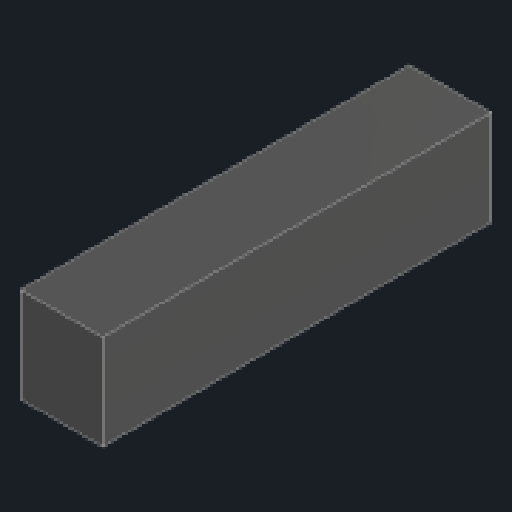
# Autodesk Inventor part: lipo2s450mah
Saved by Autodesk Inventor 2023 (Build 270158000, 158)
## iProperties
Created: 2024-05-25
Part Number: lipo2s450mah
Material: Generic
Document SubType Name: Modeling
Designer: szymo
Density: 2.33479 g/cm^3
Appearance: Dark Gray
Mass: 28 g
Surface Area: 38.34 cm^2
Volume: 11.9925 cm^3
Author: szymo
Autodesk Inventor part; units mm, degrees
ref_plane "YZ Plane" through (0, 0, 0) normal (1, 0, 0) x (0, 1, 0)
ref_plane "XZ Plane" through (0, 0, 0) normal (0, 1, 0) x (-1, 0, 0)
ref_plane "XY Plane" through (0, 0, 0) normal (0, 0, 1) x (1, 0, 0)
sketch "Sketch1" plane through (0, 0, 0) normal (0, 1, 0) x (-1, 0, 0)
  line L0 (0, 0) -> (-13, 0)
  line L1 (-13, 0) -> (-13, -61.5)
  line L2 (-13, -61.5) -> (0, -61.5)
  line L3 (0, -61.5) -> (0, 0)
  dimension "d0" = 13
  dimension "d1" = 61.5
  constraints: 8 end point, 2 parallel, 1 horizontal, 1 perpendicular
  measures "d0" distance of L2.end L1.end
  measures "d1" distance of L1.end L0.end
extrude "Extrusion1" add sketch "Sketch1" along normal blind 15
body "Solid1"
